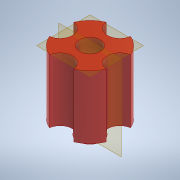
# Autodesk Inventor part: wheel spacer for bearing
Saved by Autodesk Inventor 2020 (Build 240168000, 168)
## iProperties
Created: 2020-02-25
Part Number: wheel spacer for bearing
Material: Generic
Document SubType Name: Modeling
Designer: ball
Density: 1 g/cm^3
Appearance: Default
Author: ball
Autodesk Inventor part; units mm, degrees
ref_plane "YZ Plane" through (0, 0, 0) normal (1, 0, 0) x (0, 1, 0)
ref_plane "XZ Plane" through (0, 0, 0) normal (0, 1, 0) x (-1, 0, 0)
ref_plane "Work Plane1" through (0, 31.6738, 0) normal (0, 1, 0) x (1, 0, 0)
sketch "Sketch2" plane through (0, 31.6738, 0) normal (0, 1, 0) x (1, 0, 0)
  circle A0 centre (0, 0) radius 4.25 projected
  arc A1 (5.0369, -11.6585) -> (-5.0369, -11.6585) centre (0, -12.319) ccw
  arc A2 (11.6585, 5.0369) -> (11.6585, -5.0369) centre (12.319, 0) ccw
  arc A3 (-5.0369, 11.6585) -> (5.0369, 11.6585) centre (0, 12.319) ccw
  arc A4 (-11.6585, -5.0369) -> (-11.6585, 5.0369) centre (-12.319, 0) ccw
  arc A5 (-11.6585, -5.0369) -> (-5.0369, -11.6585) centre (0, 0) ccw
  arc A6 (-5.0369, 11.6585) -> (-11.6585, 5.0369) centre (0, 0) ccw
  arc A7 (5.0369, -11.6585) -> (11.6585, -5.0369) centre (0, 0) ccw
  arc A8 (11.6585, 5.0369) -> (5.0369, 11.6585) centre (0, 0) ccw
  circle A9 centre (0, 0) radius 4.25
  dimension "d5" = 10.16
  dimension "d6" = 12.319
  dimension "d9" = 360
  constraints: 16 point on circle, 9 centre point, 2 coincident, 1 concentric, 17 other
  measures "d5" diameter of A1
  measures "d6" distance of point (0, 0) A1.centre
extrude "Extrusion2" add sketch "Sketch2" against normal blind 26.0096
sketch "Sketch3" plane through (0, 5.6642, 0) normal (0, -1, 0) x (1, 0, 0)
  circle A0 centre (0, 0) radius 4.25
  circle A1 centre (0, 0) radius 5.0038
  dimension "d13" = 10.0076
  constraints: 2 centre point, 2 coincident
  measures "d13" diameter of A1
extrude "Extrusion3" add sketch "Sketch3" along normal blind 5.6642
body "Solid1"
